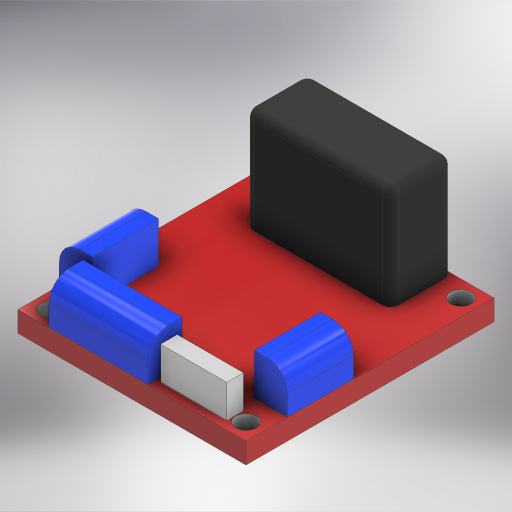
# Autodesk Inventor part: Puente H
Saved by Autodesk Inventor 2024 (Build 280153000, 153)
## iProperties
Created: 2023-11-02
Part Number: Puente H
Material: Genérico
Document SubType Name: Modeling
Designer: juesr
Density: 1 g/cm^3
Appearance: Valor por defecto
Author: juesr
Autodesk Inventor part; units mm, degrees
ref_plane "YZ Plane" through (0, 0, 0) normal (1, 0, 0) x (0, 1, 0)
ref_plane "XZ Plane" through (0, 0, 0) normal (0, 1, 0) x (-1, 0, 0)
ref_plane "XY Plane" through (0, 0, 0) normal (0, 0, 1) x (1, 0, 0)
sketch "Boceto1" plane through (0, 0, 0) normal (0, 1, 0) x (-1, 0, 0)
  line L0 (27.559, 29.972) -> (-27.559, 29.972)
  line L1 (-27.559, 29.972) -> (-27.559, -29.972)
  line L2 (-27.559, -29.972) -> (27.559, -29.972)
  line L3 (27.559, -29.972) -> (27.559, 29.972)
  point P0 (0, 0)
  point P1 (0, -29.972)
  point P2 (0, 29.972)
  dimension "d0" = 59.944
  dimension "d1" = 55.118
  dimension "d44" = 29.972
  dimension "d45" = 27.559
  constraints: 8 end point, 2 midpoint, 2 parallel, 1 horizontal, 1 perpendicular
  measures "d0" distance of point (0, -29.972) point (0, 29.972)
  measures "d1" distance between parallel lines of L1 L3
  measures "d44" distance of point (0, -29.972) point (0, 0)
  measures "d45" distance from line of L3 point (0, 0)
extrude "Extrusión1" add sketch "Boceto1" along normal blind 5
sketch "Boceto2" plane through (0, 5, 0) normal (0, 1, 0) x (1, 0, 0)
  line L0 (27.559, 29.972) -> (-27.559, 29.972) projected
  line L1 (-17.559, 29.972) -> (17.559, 29.972)
  line L2 (17.559, 29.972) -> (17.559, 14.972)
  line L3 (17.559, 14.972) -> (-17.559, 14.972)
  line L4 (-17.559, 14.972) -> (-17.559, 29.972)
  line L5 (-27.559, 29.972) -> (-27.559, -29.972) projected
  line L6 (27.559, -29.972) -> (27.559, 29.972) projected
  point P0 (0, 0)
  point P1 (17.559, 22.472)
  point P2 (17.559, 29.972)
  dimension "d4" = 10
  dimension "d5" = 10
  dimension "d6" = 15
  constraints: 8 end point, 2 parallel, 1 horizontal, 1 midpoint, 1 perpendicular, 1 point on line
  measures "d4" distance between parallel lines of L5 L4
  measures "d5" distance from line of L6 point (17.559, 22.472)
  measures "d6" distance between parallel lines of L0 L3
extrude "Extrusión2" add sketch "Boceto2" along normal blind 24.972
sketch "Boceto3" plane through (0, 5, 0) normal (0, 1, 0) x (1, 0, 0)
  line L0 (-27.559, -29.972) -> (27.559, -29.972) projected
  line L1 (-20.059, -29.972) -> (3.941, -29.972)
  line L2 (3.941, -29.972) -> (3.941, -21.7462)
  line L3 (3.941, -21.7462) -> (-20.059, -21.7462)
  line L4 (-20.059, -21.7462) -> (-20.059, -29.972)
  line L5 (-27.559, 29.972) -> (-27.559, -29.972) projected
  line L6 (-27.559, -19.972) -> (-19.559, -19.972)
  line L7 (-19.559, -19.972) -> (-19.559, -3.972)
  line L8 (-19.559, -3.972) -> (-27.559, -3.972)
  line L9 (-27.559, -3.972) -> (-27.559, -19.972)
  line L10 (27.559, -29.972) -> (27.559, 29.972) projected
  line L11 (27.559, -19.972) -> (19.559, -19.972)
  line L12 (19.559, -19.972) -> (19.559, -3.972)
  line L13 (19.559, -3.972) -> (27.559, -3.972)
  line L14 (27.559, -3.972) -> (27.559, -19.972)
  point P0 (0, 0)
  point P1 (-23.559, -19.972)
  point P2 (-20.059, -25.8591)
  point P3 (23.559, -19.972)
  point P4 (3.941, -29.972)
  dimension "d9" = 10
  dimension "d10" = 7.5
  dimension "d11" = 8
  dimension "d12" = 16
  dimension "d13" = 10
  dimension "d14" = 8
  dimension "d15" = 24
  constraints: 24 end point, 6 parallel, 4 point on line, 3 horizontal, 3 midpoint, 3 perpendicular
  measures "d9" distance from line of L0 point (-23.559, -19.972)
  measures "d10" distance from line of L5 point (-20.059, -25.859)
  measures "d11" distance between parallel lines of L5 L7
  measures "d12" distance between parallel lines of L8 L6
  measures "d13" distance from line of L0 point (23.559, -19.972)
  measures "d14" distance between parallel lines of L14 L12
  measures "d15" distance between parallel lines of L2 L4
extrude "Extrusión3" add sketch "Boceto3" along normal blind 10
sketch "Boceto4" plane through (0, 5, 0) normal (0, 1, 0) x (1, 0, 0)
  line L0 (4.941, -23.972) -> (20.941, -23.972)
  line L1 (20.941, -23.972) -> (20.941, -27.972)
  line L2 (20.941, -27.972) -> (4.941, -27.972)
  line L3 (4.941, -27.972) -> (4.941, -23.972)
  line L4 (3.941, -29.972) -> (27.559, -29.972) projected
  line L5 (3.941, -29.972) -> (3.941, -21.7462) projected
  point P0 (0, 0)
  point P1 (20.941, -25.972)
  point P2 (4.941, -25.972)
  point P3 (3.941, -25.8591)
  dimension "d18" = 2
  dimension "d19" = 4
  dimension "d20" = 16
  dimension "d21" = 1
  constraints: 8 end point, 3 midpoint, 2 parallel, 1 horizontal, 1 perpendicular
  measures "d18" distance between parallel lines of L4 L2
  measures "d19" distance between parallel lines of L2 L0
  measures "d20" distance of point (20.941, -25.972) point (4.941, -25.972)
  measures "d21" horizontal distance of point (3.941, -25.859) point (4.941, -25.972)
extrude "Extrusión4" add sketch "Boceto4" along normal blind 8
fillet "Empalme1" radius 2 1 edges at (0, 29.972, -14.972)
fillet "Empalme2" radius 2 3 edges at (-17.559, 16.486, -14.972) (-17.559, 29.3862, -15.5578) (-17.559, 29.972, -23.472)
fillet "Empalme3" radius 2 3 edges at (17.559, 16.486, -14.972) (17.559, 29.3862, -15.5578) (17.559, 29.972, -23.472)
fillet "Empalme4" radius 2 5 edges at (0, 29.972, -29.972) (-16.9732, 29.3862, -29.972) (-17.559, 16.486, -29.972) (16.9732, 29.3862, -29.972) (17.559, 16.486, -29.972)
fillet "Empalme5" radius 5 1 edges at (-27.559, 15, 11.972)
fillet "Empalme6" radius 5 1 edges at (-8.059, 15, 29.972)
fillet "Empalme7" radius 5 1 edges at (27.559, 15, 11.972)
sketch "Boceto6" plane through (27.559, 0, -29.972) normal (0, 0, -1) x (-1, 0, 0)
  line L0 (12, 27.972) -> (12, 5) projected
  line L1 (47.618, 5) -> (23.618, 5) projected
  line L2 (12, 27.972) -> (43.118, 27.972)
  line L3 (43.118, 27.972) -> (43.118, 5)
  line L4 (43.118, 5) -> (12, 5)
  line L5 (12, 5) -> (12, 27.972)
  line L6 (43.118, 27.972) -> (43.118, 5) projected
  point P0 (27.559, 0)
  point P1 (12, 5)
  dimension "d31" = 0
  constraints: 8 end point, 2 parallel, 1 horizontal, 1 perpendicular, 1 point on line
  measures "d31" distance between parallel lines of L3 L6
extrude "Extrusión5" add sketch "Boceto6" along normal blind 0.001
sketch "Boceto7" plane through (-27.559, 0, -29.972) normal (-1, 0, 0) x (0, 0, 1)
  line L0 (33.944, 5) -> (33.944, 15) projected
  line L1 (33.944, 5) -> (49.944, 5) projected
  line L2 (33.944, 10) -> (49.944, 10)
  line L3 (49.944, 10) -> (49.944, 5)
  line L4 (49.944, 5) -> (33.944, 5)
  line L5 (33.944, 5) -> (33.944, 10)
  point P0 (29.972, 0)
  constraints: 8 end point, 2 parallel, 1 horizontal, 1 midpoint, 1 perpendicular
extrude "Extrusión6" add sketch "Boceto7" along normal blind 0.001
sketch "Boceto8" plane through (-27.559, 0, 29.972) normal (0, 0, 1) x (1, 0, 0)
  line L0 (7.5, 5) -> (7.5, 15) projected
  line L1 (43.118, 5) -> (12, 5) projected
  line L2 (7.5, 10) -> (31.5, 10)
  line L3 (31.5, 10) -> (31.5, 5)
  line L4 (31.5, 5) -> (7.5, 5)
  line L5 (7.5, 5) -> (7.5, 10)
  line L6 (31.5, 5) -> (31.5, 10) projected
  point P0 (27.559, 0)
  point P1 (12, 5)
  dimension "d36" = 0
  constraints: 8 end point, 2 parallel, 1 horizontal, 1 midpoint, 1 perpendicular, 1 point on line
  measures "d36" distance between parallel lines of L3 L6
extrude "Extrusión7" add sketch "Boceto8" along normal blind 0.001
sketch "Boceto9" plane through (27.559, 0, 29.972) normal (1, 0, 0) x (0, 0, -1)
  line L0 (10, 5) -> (10, 15) projected
  line L1 (26, 5) -> (10, 5) projected
  line L2 (10, 10) -> (26, 10)
  line L3 (26, 10) -> (26, 5)
  line L4 (26, 5) -> (10, 5)
  line L5 (10, 5) -> (10, 10)
  point P0 (29.972, 0)
  constraints: 8 end point, 2 parallel, 1 horizontal, 1 midpoint, 1 perpendicular
extrude "Extrusión8" add sketch "Boceto9" along normal blind 0.001
sketch "Boceto10" plane through (0, 5, 0) normal (0, 1, 0) x (1, 0, 0)
  circle A0 centre (-23.559, 25.972) radius 2.5
  line L0 (-27.559, 29.972) -> (-27.559, -3.972) projected
  line L1 (-15.559, 29.972) -> (-27.559, 29.972) projected
  line L2 (0, 36.742) -> (0, -44.1649)
  line L3 (-51.3406, 0) -> (46.1301, 0)
  circle A1 centre (23.559, 25.972) radius 2.5
  circle A2 centre (-23.559, -25.972) radius 2.5
  line L4 (-27.559, -29.972) -> (-27.559, 3.972)
  circle A3 centre (23.559, -25.972) radius 2.5
  point P0 (0, 0)
  point P1 (27.559, 29.972)
  dimension "d41" = 5
  dimension "d42" = 4
  dimension "d43" = 4
  constraints: 6 end point, 6 symmetric about line, 4 centre point, 1 horizontal, 1 vertical, 3 other
  measures "d41" diameter of A0
  measures "d42" distance from line of L0 A0.centre
  measures "d43" distance from line of L1 A0.centre
extrude "Extrusión9" cut sketch "Boceto10" against normal blind 5
